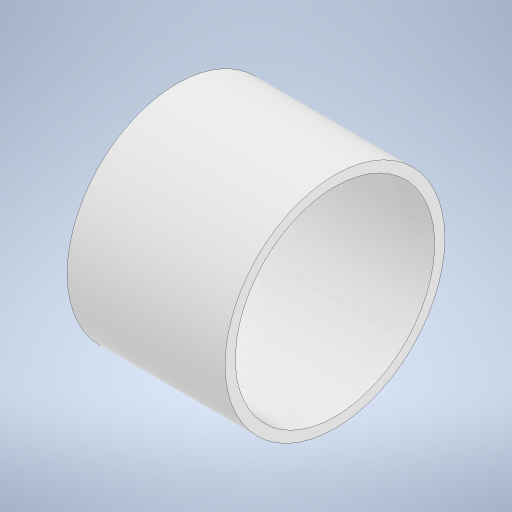
# Autodesk Inventor part: PVC Pipe
Saved by Autodesk Inventor 2023 (Build 270158030, 158C)
## iProperties
Created: 2022-09-17
Part Number: PVC Pipe
Material: PVC-Piping
Document SubType Name: Modeling
Designer: cjj5381
Density: 1.4 g/cm^3
Appearance: Smooth - White
Author: cjj5381
Autodesk Inventor part; units mm, degrees
ref_plane "YZ Plane" through (0, 0, 0) normal (1, 0, 0) x (0, 1, 0)
ref_plane "XZ Plane" through (0, 0, 0) normal (0, 1, 0) x (-1, 0, 0)
ref_plane "XY Plane" through (0, 0, 0) normal (0, 0, 1) x (1, 0, 0)
sketch "Sketch1" plane through (0, 0, 0) normal (1, 0, 0) x (0, 1, 0)
  circle A0 centre (0, 0) radius 64.0969
  circle A1 centre (0, 0) radius 70.6501
  dimension "d0" = 128.1938
  dimension "d1" = 6.5532
  constraints: 2 centre point, 1 coincident
  measures "d0" diameter of A0
  measures "d1" radial gap between concentric circles of A0 A1
extrude "Extrusion1" add sketch "Sketch1" along normal mid plane 101.6
body "Solid1"
